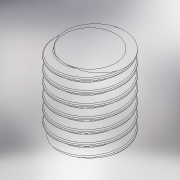
# Autodesk Inventor part: Worm
Saved by Autodesk Inventor 2019.4 (Build 234330000, 330)
## iProperties
Created: 2017-09-21
Part Number: Worm
Material: Steel, Carbon
Document SubType Name: Modeling
Designer: Ilija
Density: 7.85 g/cm^3
Appearance: Semi-Polished
Mass: 150.558 g
Surface Area: 58.8106 cm^2
Volume: 19.1794 cm^3
Sending System: SolidWorks 2017
Last Author: Ilija
Last Saved: 2017-09-27
PitchDiam: 25.000 mm
WholeDepth: 3.375 mm
LeadAngle: 3.43 deg
NormalPressureAngle: 20.00 deg
PressureAngle: 20.03 deg
ToothRatio: 0.500 ul
Starts: 1.000 ul
Module: 1.500 mm
FaceWidth: 30.000 mm
Author: Ilija
Autodesk Inventor part; units mm, degrees
ref_plane "YZ Plane" through (0, 0, 0) normal (1, 0, 0) x (0, 1, 0)
ref_plane "XZ Plane" through (0, 0, 0) normal (0, 1, 0) x (-1, 0, 0)
ref_plane "XY Plane" through (0, 0, 0) normal (0, 0, 1) x (1, 0, 0)
sketch "Sketch6" plane through (0, 0, 0) normal (1, 0, 0) x (0, 1, 0)
  line L0 (0, 0) -> (10.625, 0)
  line L1 (10.625, 0) -> (14, -0.2953)
  line L2 (14, -0.2953) -> (14, -29.7047)
  line L3 (14, -29.7047) -> (10.625, -30)
  line L4 (10.625, -30) -> (0, -30)
  line L5 (0, -30) -> (0, 0)
  dimension "d23" = 14
  dimension "d27" = 30
  dimension "d45" = 5
  dimension "d46" = 5
  dimension "d47" = 10.625
  constraints: 12 end point, 2 horizontal, 2 point on line, 1 equal length, 1 perpendicular, 1 vertical
  measures "d23" distance from line of point (0, 0) L2
  measures "d27" distance of L3.end L0.end
  measures "d45" angle of L3 L4
  measures "d46" angle of L0 L1
  measures "d47" distance of L0.start L0.end
revolve "Revolution1" add sketch "Sketch6" angle 360 about axis through (0, 0, -30) along (0, 0, 1)
sketch "Sketch5" plane through (0, 0, 0) normal (1, 0, 0) x (0, 1, 0)
  line L0 (14, 0) -> (14, 1.3801) construction
  line L1 (13.6713, 1.0323) -> (10.9537, 2.0232)
  line L2 (10.625, 2.4929) -> (10.625, 2.782)
  line L3 (10.9537, 3.2518) -> (13.6713, 4.2426)
  line L4 (12.5, 1.4594) -> (12.5, 3.8156) construction
  line L5 (14, 0.5625) -> (14, 4.7124)
  line L6 (-10.625, 0) -> (10.625, 0) projected
  arc A0 (10.9537, 3.2518) -> (10.625, 2.782) centre (11.125, 2.782) ccw
  arc A1 (10.625, 2.4929) -> (10.9537, 2.0232) centre (11.125, 2.4929) ccw
  arc A2 (13.6713, 4.2426) -> (14, 4.7124) centre (13.5, 4.7124) ccw
  arc A3 (14, 0.5625) -> (13.6713, 1.0323) centre (13.5, 0.5625) ccw
  point P0 (0, 0)
  point P1 (10.625, 2.143)
  point P2 (10.625, 3.1319)
  dimension "d10" = 40.066
  dimension "d11" = 12.5
  dimension "d12" = 10.625
  dimension "d14" = 2.3562
  dimension "d29" = 14
  dimension "d42" = 0.5
  dimension "d43" = 4.7124
  dimension "d44" = 0.5
  constraints: 12 end point, 8 point on circle, 8 tangent, 7 point on line, 4 centre point, 3 vertical, 2 equal radius, 1 collinear, 1 equal length, 1 parallel
  measures "d10" angle of L1 L3
  measures "d11" distance from line of point (0, 0) L4
  measures "d12" distance from line of point (0, 0) L2
  measures "d14" distance of L4.start L4.end
  measures "d29" distance from line of point (0, 0) L5
  measures "d42" radius of A0
  measures "d43" distance of L5.end L0.start
  measures "d44" radius of A2
coil "Coil1" sketch "Sketch5" operation cut axis through (0, 0, -10) along (0, 0, -1) pitch 4.7124 turns 7.366198 hand right
pattern_of_one "Circular Pattern1"
equation "\"d23\" = 0.5 * OuterDiam"
equation "\"d27\" = FaceWidth"
equation "\"d47\" = 0.5 * RootDiam"
equation "\"d10\" = 2 * PressureAngle"
equation "\"d11\" = 0.5 * PitchDiam"
equation "\"d12\" = 0.5 * RootDiam"
equation "\"d29\" = 0.5 * OuterDiam"
equation "\"d43\" = 3.14159 * Module"
equation "\"d16\" = 3.14159 * Module + FaceWidth"
equation "\"Starts\" = 1"
equation "\"Module\" = 1.5"
equation "\"PitchDiam\" = 25"
equation "\"OuterDiam\" = PitchDiam + 2 * Module"
equation "\"RootDiam\" = OuterDiam - 2 * WholeDepth"
equation "\"WholeDepth\" = 2.25 * Module"
equation "\"FaceWidth\" = 30"
equation "\"NormalPressureAngle\" = 20deg"
equation "\"ToothRatio\" = 0.5"
equation "\"PressureAngle\" = 20.033109deg"
body "Solid1"
body "Solid2"
